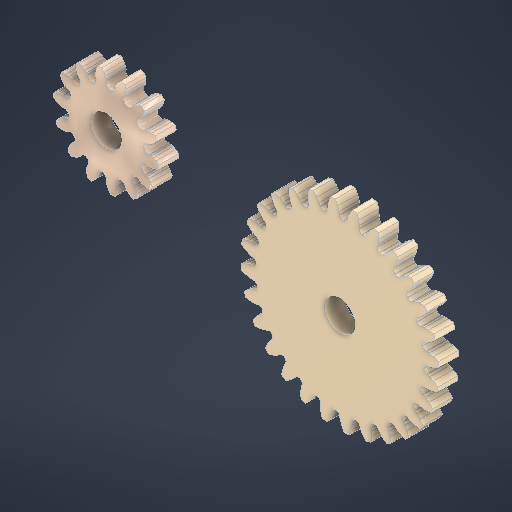
# Autodesk Inventor part: tool_kit
Saved by Autodesk Inventor 2025.3 (Build 293356030, 356C)
## iProperties
Created: 2025-09-03
Part Number: tool_kit
Material: 一般
Document SubType Name: Modeling
Designer: 陳泓任
Density: 1 g/cm^3
Appearance: 一般
Author: 陳泓任
Autodesk Inventor part; units mm, degrees
(part 1 of 2)
ref_plane "YZ Plane" through (0, 0, 0) normal (1, 0, 0) x (0, 1, 0)
ref_plane "XZ Plane" through (0, 0, 0) normal (0, 1, 0) x (-1, 0, 0)
ref_plane "XY Plane" through (0, 0, 0) normal (0, 0, 1) x (1, 0, 0)
sketch "草圖2" plane through (0, 0, 0) normal (0, 0, 1) x (1, 0, 0)
  circle A0 centre (-7.2557, 10.9657) radius 2.34
  arc A1 (-2.6311, 4.4378) -> (-2.6735, 4.985) centre (-7.0202, 4.3731) ccw
  arc A2 (-2.6735, 4.985) -> (-2.7674, 5.4236) centre (-5.8615, 4.5318) ccw
  arc A3 (-2.7674, 5.4236) -> (-2.877, 5.7246) centre (-4.9818, 4.7877) ccw
  arc A4 (-2.877, 5.7246) -> (-2.9667, 5.8946) centre (-4.149, 5.1618) ccw
  arc A5 (-2.9667, 5.8946) -> (-3.0034, 5.9471) centre (-3.4078, 5.6255) ccw
  line L0 (-3.0034, 5.9471) -> (-3.0081, 5.9526)
  arc A6 (-2.1124, 6.8641) -> (-3.0081, 5.9526) centre (-2.6737, 6.5198) ccw
  arc A7 (-2.1124, 6.8641) -> (-2.0593, 6.8294) centre (-1.8035, 7.2782) ccw
  arc A8 (-2.0593, 6.8294) -> (-1.8867, 6.7447) centre (-1.362, 8.0329) ccw
  arc A9 (-1.8867, 6.7447) -> (-1.5826, 6.6441) centre (-1.0129, 8.8764) ccw
  arc A10 (-1.5826, 6.6441) -> (-1.1415, 6.5633) centre (-0.7832, 9.7634) ccw
  arc A11 (-1.1415, 6.5633) -> (-0.5932, 6.5372) centre (-0.659, 10.9263) ccw
  arc A12 (-0.2567, 7.0908) -> (-0.5324, 7.5655) centre (-4.1831, 5.1281) ccw
  arc A13 (-0.5324, 7.5655) -> (-0.8072, 7.9198) centre (-3.208, 5.7739) ccw
  arc A14 (-0.8072, 7.9198) -> (-1.0366, 8.1435) centre (-2.5264, 6.3861) ccw
  arc A15 (-1.0366, 8.1435) -> (-1.1912, 8.2577) centre (-1.9384, 7.0845) ccw
  arc A16 (-1.1912, 8.2577) -> (-1.247, 8.2891) centre (-1.4718, 7.8239) ccw
  line L1 (-1.247, 8.2891) -> (-1.2536, 8.292)
  arc A17 (-0.8422, 9.5019) -> (-1.2536, 8.292) centre (-1.1985, 8.9482) ccw
  arc A18 (-0.8422, 9.5019) -> (-0.7792, 9.4936) centre (-0.7435, 10.009) ccw
  arc A19 (-0.7792, 9.4936) -> (-0.587, 9.4922) centre (-0.6731, 10.8805) ccw
  arc A20 (-0.587, 9.4922) -> (-0.2694, 9.5335) centre (-0.7246, 11.792) ccw
  arc A21 (-0.2694, 9.5335) -> (0.1632, 9.6521) centre (-0.9025, 12.6907) ccw
  arc A22 (0.1632, 9.6521) -> (0.6684, 9.8665) centre (-1.2952, 13.7924) ccw
  arc A23 (0.7314, 10.5113) -> (0.2771, 10.8193) centre (-1.9546, 7.0394) ccw
  arc A24 (0.2771, 10.8193) -> (-0.1243, 11.0193) centre (-1.3562, 8.0443) ccw
  arc A25 (-0.1243, 11.0193) -> (-0.4279, 11.1213) centre (-1.0078, 8.8916) ccw
  arc A26 (-0.4279, 11.1213) -> (-0.6168, 11.1571) centre (-0.781, 9.7759) ccw
  arc A27 (-0.6168, 11.1571) -> (-0.6807, 11.1612) centre (-0.6814, 10.6445) ccw
  line L2 (-0.6807, 11.1612) -> (-0.6879, 11.161)
  arc A28 (-0.8422, 12.4296) -> (-0.6879, 11.161) centre (-0.923, 11.7761) ccw
  arc A29 (-0.8422, 12.4296) -> (-0.7819, 12.4494) centre (-0.9733, 12.9293) ccw
  arc A30 (-0.7819, 12.4494) -> (-0.6081, 12.5316) centre (-1.288, 13.745) ccw
  arc A31 (-0.6081, 12.5316) -> (-0.3398, 12.7066) centre (-1.7299, 14.5439) ccw
  arc A32 (-0.3398, 12.7066) -> (-0.0016, 13.0011) centre (-2.2801, 15.2764) ccw
  arc A33 (-0.0016, 13.0011) -> (0.3606, 13.4135) centre (-3.1119, 16.0986) ccw
  arc A34 (0.1376, 14.0217) -> (-0.4053, 14.1022) centre (-0.776, 9.7283) ccw
  arc A35 (-0.4053, 14.1022) -> (-0.8538, 14.1082) centre (-0.6729, 10.8933) ccw
  arc A36 (-0.8538, 14.1082) -> (-1.1716, 14.0684) centre (-0.7266, 11.8079) ccw
  arc A37 (-1.1716, 14.0684) -> (-1.3573, 14.0187) centre (-0.906, 12.703) ccw
  arc A38 (-1.3573, 14.0187) -> (-1.4167, 13.9946) centre (-1.1931, 13.5288) ccw
  line L3 (-1.4167, 13.9946) -> (-1.4231, 13.9913)
  arc A39 (-2.1125, 15.0673) -> (-1.4231, 13.9913) centre (-1.9017, 14.4435) ccw
  arc A40 (-2.1125, 15.0673) -> (-2.0667, 15.1114) centre (-2.4474, 15.4607) ccw
  arc A41 (-2.0667, 15.1114) -> (-1.9458, 15.2608) centre (-3.0849, 16.059) ccw
  arc A42 (-1.9458, 15.2608) -> (-1.7801, 15.5349) centre (-3.8296, 16.5871) ccw
  arc A43 (-1.7801, 15.5349) -> (-1.6031, 15.947) centre (-4.6432, 17.0083) ccw
  arc A44 (-1.6031, 15.947) -> (-1.4557, 16.4757) centre (-5.7494, 17.3882) ccw
  arc A45 (-1.9205, 16.9269) -> (-2.4446, 16.7638) centre (-0.8808, 12.6622) ccw
  arc A46 (-2.4446, 16.7638) -> (-2.8513, 16.5747) centre (-1.2934, 13.7566) ccw
  arc A47 (-2.8513, 16.5747) -> (-3.1203, 16.4009) centre (-1.7386, 14.5573) ccw
  arc A48 (-3.1203, 16.4009) -> (-3.2661, 16.2756) centre (-2.2886, 15.286) ccw
  arc A49 (-3.2661, 16.2756) -> (-3.3091, 16.2281) centre (-2.9056, 15.9054) ccw
  line L4 (-3.3091, 16.2281) -> (-3.3134, 16.2223)
  arc A50 (-4.4014, 16.8927) -> (-3.3134, 16.2223) centre (-3.9409, 16.4221) ccw
  arc A51 (-4.4014, 16.8927) -> (-4.3793, 16.9522) centre (-4.8739, 17.1018) ccw
  arc A52 (-4.3793, 16.9522) -> (-4.3352, 17.1393) centre (-5.7078, 17.3643) ccw
  arc A53 (-4.3352, 17.1393) -> (-4.3048, 17.4582) centre (-6.6079, 17.5169) ccw
  arc A54 (-4.3048, 17.4582) -> (-4.3242, 17.9062) centre (-7.5237, 17.5434) ccw
  arc A55 (-4.3242, 17.9062) -> (-4.4207, 18.4466) centre (-8.6852, 17.4058) ccw
  arc A56 (-5.0353, 18.6514) -> (-5.4368, 18.2771) centre (-2.2482, 15.2602) ccw
  arc A57 (-5.4368, 18.2771) -> (-5.7211, 17.9302) centre (-3.0947, 16.0672) ccw
  arc A58 (-5.7211, 17.9302) -> (-5.8881, 17.6569) centre (-3.8433, 16.5954) ccw
  arc A59 (-5.8881, 17.6569) -> (-5.965, 17.4808) centre (-4.655, 17.0133) ccw
  arc A60 (-5.965, 17.4808) -> (-5.9832, 17.4193) centre (-5.4796, 17.3037) ccw
  line L5 (-5.9832, 17.4193) -> (-5.9846, 17.4123)
  arc A61 (-7.2557, 17.5441) -> (-5.9846, 17.4123) centre (-6.6366, 17.32) ccw
  arc A62 (-7.2557, 17.5441) -> (-7.2616, 17.6074) centre (-7.7721, 17.5275) ccw
  arc A63 (-7.2616, 17.6074) -> (-7.3031, 17.7951) centre (-8.6374, 17.4022) ccw
  arc A64 (-7.3031, 17.7951) -> (-7.414, 18.0956) centre (-9.5146, 17.1492) ccw
  arc A65 (-7.414, 18.0956) -> (-7.6259, 18.4908) centre (-10.3512, 16.7757) ccw
  arc A66 (-7.6259, 18.4908) -> (-7.9473, 18.9358) centre (-11.3378, 16.1478) ccw
  arc A67 (-8.5899, 18.8537) -> (-8.7892, 18.3422) centre (-4.6074, 17.0076) ccw
  arc A68 (-8.7892, 18.3422) -> (-8.8949, 17.9064) centre (-5.7202, 17.3673) ccw
  arc A69 (-8.8949, 17.9064) -> (-8.9267, 17.5876) centre (-6.6239, 17.5185) ccw
  arc A70 (-8.9267, 17.5876) -> (-8.9196, 17.3956) centre (-7.5365, 17.5428) ccw
  arc A71 (-8.9196, 17.3956) -> (-8.9093, 17.3323) centre (-8.4055, 17.4466) ccw
  line L6 (-8.9093, 17.3323) -> (-8.9075, 17.3253)
  arc A72 (-10.11, 16.8927) -> (-8.9075, 17.3253) centre (-9.4549, 16.9593) ccw
  arc A73 (-10.11, 16.8927) -> (-10.1428, 16.947) centre (-10.568, 16.6536) ccw
  arc A74 (-10.1428, 16.947) -> (-10.2615, 17.0982) centre (-11.2932, 16.1653) ccw
  arc A75 (-10.2615, 17.0982) -> (-10.4919, 17.3208) centre (-11.9738, 15.5567) ccw
  arc A76 (-10.4919, 17.3208) -> (-10.8543, 17.585) centre (-12.5655, 14.8573) ccw
  arc A77 (-10.8543, 17.585) -> (-11.3369, 17.8464) centre (-13.182, 13.8634) ccw
  arc A78 (-11.8803, 17.4936) -> (-11.8379, 16.9464) centre (-7.4911, 17.5583) ccw
  arc A79 (-11.8379, 16.9464) -> (-11.744, 16.5078) centre (-8.6499, 17.3996) ccw
  arc A80 (-11.744, 16.5078) -> (-11.6344, 16.2068) centre (-9.5296, 17.1437) ccw
  arc A81 (-11.6344, 16.2068) -> (-11.5446, 16.0368) centre (-10.3624, 16.7696) ccw
  arc A82 (-11.5446, 16.0368) -> (-11.5079, 15.9843) centre (-11.1036, 16.3059) ccw
  line L7 (-11.5079, 15.9843) -> (-11.5033, 15.9788)
  arc A83 (-12.3989, 15.0673) -> (-11.5033, 15.9788) centre (-11.8376, 15.4116) ccw
  arc A84 (-12.3989, 15.0673) -> (-12.4521, 15.1021) centre (-12.7079, 14.6532) ccw
  arc A85 (-12.4521, 15.1021) -> (-12.6246, 15.1867) centre (-13.1494, 13.8985) ccw
  arc A86 (-12.6246, 15.1867) -> (-12.9288, 15.2873) centre (-13.4985, 13.055) ccw
  arc A87 (-12.9288, 15.2873) -> (-13.3699, 15.3681) centre (-13.7281, 12.168) ccw
  arc A88 (-13.3699, 15.3681) -> (-13.9181, 15.3942) centre (-13.8524, 11.0051) ccw
  arc A89 (-14.2546, 14.8406) -> (-13.979, 14.366) centre (-10.3282, 16.8033) ccw
  arc A90 (-13.979, 14.366) -> (-13.7041, 14.0116) centre (-11.3033, 16.1575) ccw
  arc A91 (-13.7041, 14.0116) -> (-13.4748, 13.7879) centre (-11.9849, 15.5453) ccw
  arc A92 (-13.4748, 13.7879) -> (-13.3202, 13.6737) centre (-12.573, 14.8469) ccw
  arc A93 (-13.3202, 13.6737) -> (-13.2643, 13.6423) centre (-13.0395, 14.1075) ccw
  line L8 (-13.2643, 13.6423) -> (-13.2578, 13.6394)
  arc A94 (-13.6692, 12.4295) -> (-13.2578, 13.6394) centre (-13.3129, 12.9832) ccw
  arc A95 (-13.6692, 12.4295) -> (-13.7321, 12.4378) centre (-13.7679, 11.9224) ccw
  arc A96 (-13.7321, 12.4378) -> (-13.9243, 12.4392) centre (-13.8382, 11.0509) ccw
  arc A97 (-13.9243, 12.4392) -> (-14.242, 12.3979) centre (-13.7868, 10.1394) ccw
  arc A98 (-14.242, 12.3979) -> (-14.6745, 12.2793) centre (-13.6088, 9.2407) ccw
  arc A99 (-14.6745, 12.2793) -> (-15.1798, 12.0649) centre (-13.2162, 8.139) ccw
  arc A100 (-15.231, 11.5938) -> (-15.2428, 11.4201) centre (-7.2557, 10.9657) ccw
  arc A101 (-15.2428, 11.4201) -> (-14.7885, 11.1121) centre (-12.5568, 14.892) ccw
  arc A102 (-14.7885, 11.1121) -> (-14.3871, 10.9121) centre (-13.1551, 13.8871) ccw
  arc A103 (-14.3871, 10.9121) -> (-14.0834, 10.8101) centre (-13.5036, 13.0398) ccw
  arc A104 (-14.0834, 10.8101) -> (-13.8946, 10.7743) centre (-13.7304, 12.1555) ccw
  arc A105 (-13.8946, 10.7743) -> (-13.8306, 10.7702) centre (-13.83, 11.2869) ccw
  line L9 (-13.8306, 10.7702) -> (-13.8235, 10.7704)
  arc A106 (-13.6692, 9.5018) -> (-13.8235, 10.7704) centre (-13.5884, 10.1553) ccw
  arc A107 (-13.6692, 9.5018) -> (-13.7295, 9.482) centre (-13.5381, 9.0021) ccw
  arc A108 (-13.7295, 9.482) -> (-13.9033, 9.3998) centre (-13.2233, 8.1864) ccw
  arc A109 (-13.9033, 9.3998) -> (-14.1715, 9.2248) centre (-12.7815, 7.3875) ccw
  arc A110 (-14.1715, 9.2248) -> (-14.5098, 8.9303) centre (-12.2312, 6.655) ccw
  arc A111 (-14.5098, 8.9303) -> (-14.872, 8.5179) centre (-11.3995, 5.8328) ccw
  arc A112 (-14.649, 7.9097) -> (-14.106, 7.8292) centre (-13.7354, 12.2032) ccw
  arc A113 (-14.106, 7.8292) -> (-13.6576, 7.8232) centre (-13.8385, 11.0382) ccw
  arc A114 (-13.6576, 7.8232) -> (-13.3397, 7.8631) centre (-13.7848, 10.1235) ccw
  arc A115 (-13.3397, 7.8631) -> (-13.1541, 7.9127) centre (-13.6054, 9.2284) ccw
  arc A116 (-13.1541, 7.9127) -> (-13.0947, 7.9368) centre (-13.3182, 8.4026) ccw
  line L10 (-13.0947, 7.9368) -> (-13.0883, 7.9401)
  arc A117 (-12.3989, 6.8641) -> (-13.0883, 7.9401) centre (-12.6097, 7.4879) ccw
  arc A118 (-12.3989, 6.8641) -> (-12.4446, 6.82) centre (-12.0639, 6.4707) ccw
  arc A119 (-12.4446, 6.82) -> (-12.5655, 6.6706) centre (-11.4265, 5.8724) ccw
  arc A120 (-12.5655, 6.6706) -> (-12.7313, 6.3965) centre (-10.6817, 5.3443) ccw
  arc A121 (-12.7313, 6.3965) -> (-12.9083, 5.9844) centre (-9.8681, 4.9231) ccw
  arc A122 (-12.9083, 5.9844) -> (-13.0557, 5.4557) centre (-8.762, 4.5432) ccw
  arc A123 (-12.5908, 5.0045) -> (-12.0668, 5.1676) centre (-13.6306, 9.2692) ccw
  arc A124 (-12.0668, 5.1676) -> (-11.6601, 5.3567) centre (-13.218, 8.1748) ccw
  arc A125 (-11.6601, 5.3567) -> (-11.391, 5.5305) centre (-12.7728, 7.3741) ccw
  arc A126 (-11.391, 5.5305) -> (-11.2453, 5.6558) centre (-12.2228, 6.6454) ccw
  arc A127 (-11.2453, 5.6558) -> (-11.2022, 5.7033) centre (-11.6058, 6.026) ccw
  line L11 (-11.2022, 5.7033) -> (-11.1979, 5.7091)
  arc A128 (-10.1099, 5.0387) -> (-11.1979, 5.7091) centre (-10.5705, 5.5093) ccw
  arc A129 (-10.1099, 5.0387) -> (-10.132, 4.9792) centre (-9.6375, 4.8296) ccw
  arc A130 (-10.132, 4.9792) -> (-10.1761, 4.7921) centre (-8.8035, 4.5672) ccw
  arc A131 (-10.1761, 4.7921) -> (-10.2066, 4.4732) centre (-7.9034, 4.4145) ccw
  arc A132 (-10.2066, 4.4732) -> (-10.1872, 4.0252) centre (-6.9876, 4.388) ccw
  arc A133 (-10.1872, 4.0252) -> (-10.0906, 3.4849) centre (-5.8262, 4.5256) ccw
  arc A134 (-9.476, 3.28) -> (-9.0746, 3.6543) centre (-12.2632, 6.6712) ccw
  arc A135 (-9.0746, 3.6543) -> (-8.7903, 4.0012) centre (-11.4166, 5.8642) ccw
  arc A136 (-8.7903, 4.0012) -> (-8.6233, 4.2745) centre (-10.6681, 5.336) ccw
  arc A137 (-8.6233, 4.2745) -> (-8.5463, 4.4507) centre (-9.8564, 4.9181) ccw
  arc A138 (-8.5463, 4.4507) -> (-8.5282, 4.5121) centre (-9.0317, 4.6277) ccw
  line L12 (-8.5282, 4.5121) -> (-8.5268, 4.5191)
  arc A139 (-7.2557, 4.3873) -> (-8.5268, 4.5191) centre (-7.8748, 4.6114) ccw
  arc A140 (-7.2557, 4.3873) -> (-7.2497, 4.324) centre (-6.7393, 4.4039) ccw
  arc A141 (-7.2497, 4.324) -> (-7.2083, 4.1364) centre (-5.874, 4.5292) ccw
  arc A142 (-7.2083, 4.1364) -> (-7.0973, 3.8358) centre (-4.9968, 4.7822) ccw
  arc A143 (-7.0973, 3.8358) -> (-6.8855, 3.4406) centre (-4.1602, 5.1557) ccw
  arc A144 (-6.8855, 3.4406) -> (-6.5641, 2.9957) centre (-3.1735, 5.7836) ccw
  arc A145 (-5.9214, 3.0778) -> (-5.7222, 3.5892) centre (-9.904, 4.9238) ccw
  arc A146 (-5.7222, 3.5892) -> (-5.6165, 4.025) centre (-8.7911, 4.5641) ccw
  arc A147 (-5.6165, 4.025) -> (-5.5847, 4.3438) centre (-7.8875, 4.4129) ccw
  arc A148 (-5.5847, 4.3438) -> (-5.5918, 4.5359) centre (-6.9749, 4.3886) ccw
  arc A149 (-5.5918, 4.5359) -> (-5.602, 4.5991) centre (-6.1059, 4.4848) ccw
  line L13 (-5.602, 4.5991) -> (-5.6038, 4.6061)
  arc A150 (-4.4014, 5.0387) -> (-5.6038, 4.6061) centre (-5.0565, 4.9721) ccw
  arc A151 (-4.4014, 5.0387) -> (-4.3686, 4.9844) centre (-3.9433, 5.2778) ccw
  arc A152 (-4.3686, 4.9844) -> (-4.2499, 4.8332) centre (-3.2182, 5.7661) ccw
  arc A153 (-4.2499, 4.8332) -> (-4.0195, 4.6106) centre (-2.5376, 6.3747) ccw
  arc A154 (-4.0195, 4.6106) -> (-3.6571, 4.3464) centre (-1.9459, 7.0741) ccw
  arc A155 (-3.6571, 4.3464) -> (-3.1745, 4.085) centre (-1.3294, 8.068) ccw
  circle A156 centre (28.1558, 4.4199) radius 2.34
  arc A157 (31.0202, 18.3926) -> (30.8085, 19.1835) centre (24.7058, 17.1262) ccw
  arc A158 (31.1028, 17.7572) -> (31.0202, 18.3926) centre (26.5033, 17.4821) ccw
  arc A159 (31.1, 17.3728) -> (31.1028, 17.7572) centre (28.3263, 17.585) ccw
  arc A160 (31.0898, 17.2827) -> (31.1, 17.3728) centre (30.0691, 17.4444) ccw
  arc A161 (31.0898, 17.2827) -> (31.4895, 16.7266) centre (31.6154, 17.2389) ccw
  line L14 (31.4895, 16.7266) -> (31.4898, 16.728)
  arc A162 (31.4898, 16.728) -> (31.5032, 16.7235) centre (31.6675, 17.2247) ccw
  arc A163 (31.5032, 16.7235) -> (31.517, 16.7206) centre (31.6154, 17.2389) ccw
  line L15 (31.517, 16.7206) -> (31.5166, 16.7192)
  arc A164 (31.5166, 16.7192) -> (32.143, 16.9961) centre (31.6675, 17.2247) ccw
  arc A165 (32.1798, 17.0791) -> (32.143, 16.9961) centre (33.1048, 16.6184) ccw
  arc A166 (32.3722, 17.4119) -> (32.1798, 17.0791) centre (34.6787, 15.8567) ccw
  arc A167 (32.7653, 17.9178) -> (32.3722, 17.4119) centre (36.1983, 14.8444) ccw
  arc A168 (33.3485, 18.4924) -> (32.7653, 17.9178) centre (37.5677, 13.6269) ccw
  arc A169 (34.0576, 17.4049) -> (34.0272, 18.2231) centre (27.6197, 17.5754) ccw
  arc A170 (33.9967, 16.7671) -> (34.0576, 17.4049) centre (29.4513, 17.5224) ccw
  arc A171 (33.9085, 16.3929) -> (33.9967, 16.7671) centre (31.2515, 17.217) ccw
  arc A172 (33.8784, 16.3073) -> (33.9085, 16.3929) centre (32.9194, 16.692) ccw
  arc A173 (33.8784, 16.3073) -> (34.1444, 15.6763) centre (34.3812, 16.1476) ccw
  line L16 (34.1444, 15.6763) -> (34.1451, 15.6775)
  arc A174 (34.1451, 15.6775) -> (34.1571, 15.6701) centre (34.4288, 16.1222) ccw
  arc A175 (34.1571, 15.6701) -> (34.1699, 15.6643) centre (34.3812, 16.1476) ccw
  line L17 (34.1699, 15.6643) -> (34.1692, 15.663)
  arc A176 (34.1692, 15.663) -> (34.8415, 15.7936) centre (34.4288, 16.1222) ccw
  arc A177 (34.8958, 15.8663) -> (34.8415, 15.7936) centre (35.6952, 15.2113) ccw
  arc A178 (35.1574, 16.1479) -> (34.8958, 15.8663) centre (37.0601, 14.1185) ccw
  arc A179 (35.6533, 16.5537) -> (35.1574, 16.1479) centre (38.3163, 12.7934) ccw
  arc A180 (36.3498, 16.9841) -> (35.6533, 16.5537) centre (39.3805, 11.3017) ccw
  arc A181 (36.799, 15.7661) -> (36.9514, 16.5705) centre (30.5605, 17.3648) ccw
  arc A182 (36.5978, 15.1578) -> (36.799, 15.7661) centre (32.3344, 16.9056) ccw
  arc A183 (36.4285, 14.8127) -> (36.5978, 15.1578) centre (34.0215, 16.2073) ccw
  arc A184 (36.3802, 14.7359) -> (36.4285, 14.8127) centre (35.5308, 15.3244) ccw
  arc A185 (36.3802, 14.7359) -> (36.499, 14.0615) centre (36.8348, 14.4683) ccw
  line L18 (36.499, 14.0615) -> (36.5, 14.0626)
  arc A186 (36.5, 14.0626) -> (36.51, 14.0526) centre (36.8756, 14.4329) ccw
  arc A187 (36.51, 14.0526) -> (36.5212, 14.0441) centre (36.8348, 14.4683) ccw
  line L19 (36.5212, 14.0441) -> (36.5203, 14.043)
  arc A188 (36.5203, 14.043) -> (37.2047, 14.0207) centre (36.8756, 14.4329) ccw
  arc A189 (37.2739, 14.0795) -> (37.2047, 14.0207) centre (37.9075, 13.2631) ccw
  arc A190 (37.5916, 14.2959) -> (37.2739, 14.0795) centre (38.995, 11.8939) ccw
  arc A191 (38.1653, 14.5811) -> (37.5916, 14.2959) centre (39.9249, 10.3226) ccw
  arc A192 (38.9401, 14.8458) -> (38.1653, 14.5811) centre (40.6304, 8.6315) ccw
  arc A193 (39.1071, 13.5583) -> (39.4347, 14.3087) centre (33.3807, 16.5052) ccw
  arc A194 (38.7755, 13.0101) -> (39.1071, 13.5583) centre (35.008, 15.6627) ccw
  arc A195 (38.5337, 12.7112) -> (38.7755, 13.0101) centre (36.4974, 14.6065) ccw
  arc A196 (38.4695, 12.6471) -> (38.5337, 12.7112) centre (37.7723, 13.4099) ccw
  arc A197 (38.4695, 12.6471) -> (38.4353, 11.9632) centre (38.8531, 12.2851) ccw
  line L20 (38.4353, 11.9632) -> (38.4364, 11.9641)
  arc A198 (38.4364, 11.9641) -> (38.444, 11.9522) centre (38.885, 12.2416) ccw
  arc A199 (38.444, 11.9522) -> (38.4531, 11.9413) centre (38.8531, 12.2851) ccw
  line L21 (38.4531, 11.9413) -> (38.4519, 11.9405)
  arc A200 (38.4519, 11.9405) -> (39.1142, 11.7665) centre (38.885, 12.2416) ccw
  arc A201 (39.1947, 11.8083) -> (39.1142, 11.7665) centre (39.6308, 10.8715) ccw
  arc A202 (39.5527, 11.9486) -> (39.1947, 11.8083) centre (40.3864, 9.2946) ccw
  arc A203 (40.1754, 12.099) -> (39.5527, 11.9486) centre (40.9433, 7.5557) ccw
  arc A204 (40.9897, 12.1847) -> (40.1754, 12.099) centre (41.2548, 5.75) ccw
  arc A205 (40.866, 10.8923) -> (41.3523, 11.551) centre (35.9389, 15.0395) ccw
  arc A206 (40.4208, 10.4316) -> (40.866, 10.8923) centre (37.3379, 13.8561) ccw
  arc A207 (40.1185, 10.1941) -> (40.4208, 10.4316) centre (38.555, 12.495) ccw
  arc A208 (40.0416, 10.1459) -> (40.1185, 10.1941) centre (39.5317, 11.0446) ccw
  arc A209 (40.0416, 10.1459) -> (39.8561, 9.4867) centre (40.3351, 9.7076) ccw
  line L22 (39.8561, 9.4867) -> (39.8574, 9.4873)
  arc A210 (39.8574, 9.4873) -> (39.8622, 9.474) centre (40.3565, 9.658) ccw
  arc A211 (39.8622, 9.474) -> (39.8686, 9.4614) centre (40.3351, 9.7076) ccw
  line L23 (39.8686, 9.4614) -> (39.8673, 9.4608)
  arc A212 (39.8673, 9.4608) -> (40.4742, 9.1438) centre (40.3565, 9.658) ccw
  arc A213 (40.5621, 9.1667) -> (40.4742, 9.1438) centre (40.7787, 8.1563) ccw
  arc A214 (40.9422, 9.2238) -> (40.5621, 9.1667) centre (41.1644, 6.4508) ccw
  arc A215 (41.5828, 9.2319) -> (40.9422, 9.2238) centre (41.3204, 4.6316) ccw
  arc A216 (42.3958, 9.1342) -> (41.5828, 9.2319) centre (41.2224, 2.8019) ccw
  arc A217 (41.9875, 7.9017) -> (42.6083, 8.4357) centre (38.1069, 13.0414) ccw
  arc A218 (41.451, 7.5516) -> (41.9875, 7.9017) centre (39.2074, 11.5763) ccw
  arc A219 (41.1034, 7.3874) -> (41.451, 7.5516) centre (40.0911, 9.9785) ccw
  arc A220 (41.0178, 7.3575) -> (41.1034, 7.3874) centre (40.7206, 8.3472) ccw
  arc A221 (41.0178, 7.3575) -> (40.6902, 6.7561) centre (41.2064, 6.8648) ccw
  line L24 (40.6902, 6.7561) -> (40.6916, 6.7564)
  arc A222 (40.6916, 6.7564) -> (40.6933, 6.7423) centre (41.2162, 6.8117) ccw
  arc A223 (40.6933, 6.7423) -> (40.6968, 6.7287) centre (41.2064, 6.8648) ccw
  line L25 (40.6968, 6.7287) -> (40.6953, 6.7284)
  arc A224 (40.6953, 6.7284) -> (41.2166, 6.2842) centre (41.2162, 6.8117) ccw
  arc A225 (41.3073, 6.287) -> (41.2166, 6.2842) centre (41.2936, 5.2538) ccw
  arc A226 (41.6906, 6.2581) -> (41.3073, 6.287) centre (41.2902, 3.5052) ccw
  arc A227 (42.3169, 6.1234) -> (41.6906, 6.2581) centre (41.0375, 1.6969) ccw
  arc A228 (43.0878, 5.8473) -> (42.3169, 6.1234) centre (40.5347, -0.0652) ccw
  arc A229 (42.4155, 4.7366) -> (43.1395, 5.119) centre (39.7758, 10.6109) ccw
  arc A230 (41.8145, 4.5147) -> (42.4155, 4.7366) centre (40.5228, 8.9377) ccw
  arc A231 (41.4391, 4.4318) -> (41.8145, 4.5147) centre (41.0288, 7.1833) ccw
  arc A232 (41.3489, 4.4218) -> (41.4391, 4.4318) centre (41.2795, 5.4528) ccw
  arc A233 (41.3489, 4.4218) -> (40.8958, 3.9084) centre (41.4232, 3.8995) ccw
  line L26 (40.8958, 3.9084) -> (40.8972, 3.9083)
  arc A234 (40.8972, 3.9083) -> (40.8957, 3.8943) centre (41.421, 3.8456) ccw
  arc A235 (40.8957, 3.8943) -> (40.8961, 3.8801) centre (41.4232, 3.8995) ccw
  line L27 (40.8961, 3.8801) -> (40.8946, 3.8802)
  arc A236 (40.8946, 3.8802) -> (41.3039, 3.3312) centre (41.421, 3.8456) ccw
  arc A237 (41.393, 3.3138) -> (41.3039, 3.3312) centre (41.1498, 2.3094) ccw
  arc A238 (41.7603, 3.2003) -> (41.393, 3.3138) centre (40.7574, 0.6055) ccw
  arc A239 (42.341, 2.9296) -> (41.7603, 3.2003) centre (40.1086, -1.1013) ccw
  arc A240 (43.031, 2.4888) -> (42.341, 2.9296) centre (39.2263, -2.7073) ccw
  arc A241 (42.1285, 1.5556) -> (42.9194, 1.7673) centre (40.8621, 7.87) ccw
  arc A242 (41.4931, 1.473) -> (42.1285, 1.5556) centre (41.218, 6.0725) ccw
  arc A243 (41.1087, 1.4757) -> (41.4931, 1.473) centre (41.3209, 4.2495) ccw
  arc A244 (41.0186, 1.486) -> (41.1087, 1.4757) centre (41.1802, 2.5066) ccw
  arc A245 (41.0186, 1.486) -> (40.4625, 1.0863) centre (40.9748, 0.9603) ccw
  line L28 (40.4625, 1.0863) -> (40.4639, 1.0859)
  arc A246 (40.4639, 1.0859) -> (40.4593, 1.0725) centre (40.9606, 0.9082) ccw
  arc A247 (40.4593, 1.0725) -> (40.4565, 1.0587) centre (40.9748, 0.9603) ccw
  line L29 (40.4565, 1.0587) -> (40.4551, 1.0591)
  arc A248 (40.4551, 1.0591) -> (40.732, 0.4328) centre (40.9606, 0.9082) ccw
  arc A249 (40.815, 0.3959) -> (40.732, 0.4328) centre (40.3543, -0.5291) ccw
  arc A250 (41.1478, 0.2036) -> (40.815, 0.3959) centre (39.5926, -2.103) ccw
  arc A251 (41.6537, -0.1895) -> (41.1478, 0.2036) centre (38.5803, -3.6226) ccw
  arc A252 (42.2283, -0.7728) -> (41.6537, -0.1895) centre (37.3628, -4.992) ccw
  arc A253 (41.1408, -1.4818) -> (41.959, -1.4514) centre (41.3113, 4.956) ccw
  arc A254 (40.503, -1.421) -> (41.1408, -1.4818) centre (41.2583, 3.1244) ccw
  arc A255 (40.1288, -1.3328) -> (40.503, -1.421) centre (40.9529, 1.3242) ccw
  arc A256 (40.0432, -1.3027) -> (40.1288, -1.3328) centre (40.4279, -0.3436) ccw
  arc A257 (40.0432, -1.3027) -> (39.4122, -1.5686) centre (39.8835, -1.8054) ccw
  line L30 (39.4122, -1.5686) -> (39.4134, -1.5693)
  arc A258 (39.4134, -1.5693) -> (39.406, -1.5813) centre (39.8581, -1.8531) ccw
  arc A259 (39.406, -1.5813) -> (39.4002, -1.5942) centre (39.8835, -1.8054) ccw
  line L31 (39.4002, -1.5942) -> (39.3989, -1.5935)
  arc A260 (39.3989, -1.5935) -> (39.5295, -2.2657) centre (39.8581, -1.8531) ccw
  arc A261 (39.6022, -2.3201) -> (39.5295, -2.2657) centre (38.9472, -3.1194) ccw
  arc A262 (39.8838, -2.5817) -> (39.6022, -2.3201) centre (37.8544, -4.4844) ccw
  arc A263 (40.2896, -3.0775) -> (39.8838, -2.5817) centre (36.5293, -5.7406) ccw
  arc A264 (40.72, -3.774) -> (40.2896, -3.0775) centre (35.0376, -6.8048) ccw
  arc A265 (39.502, -4.2233) -> (40.3064, -4.3757) centre (41.1007, 2.0152) ccw
  arc A266 (38.8937, -4.0221) -> (39.502, -4.2233) centre (40.6415, 0.2413) ccw
  arc A267 (38.5486, -3.8528) -> (38.8937, -4.0221) centre (39.9432, -1.4458) ccw
  arc A268 (38.4718, -3.8044) -> (38.5486, -3.8528) centre (39.0603, -2.955) ccw
  arc A269 (38.4718, -3.8044) -> (37.7974, -3.9233) centre (38.2042, -4.259) ccw
  line L32 (37.7974, -3.9233) -> (37.7985, -3.9242)
  arc A270 (37.7985, -3.9242) -> (37.7885, -3.9343) centre (38.1688, -4.2998) ccw
  arc A271 (37.7885, -3.9343) -> (37.78, -3.9455) centre (38.2042, -4.259) ccw
  line L33 (37.78, -3.9455) -> (37.7789, -3.9446)
  arc A272 (37.7789, -3.9446) -> (37.7566, -4.629) centre (38.1688, -4.2998) ccw
  arc A273 (37.8154, -4.6982) -> (37.7566, -4.629) centre (36.999, -5.3317) ccw
  arc A274 (38.0318, -5.0159) -> (37.8154, -4.6982) centre (35.6298, -6.4193) ccw
  arc A275 (38.317, -5.5896) -> (38.0318, -5.0159) centre (34.0585, -7.3491) ccw
  arc A276 (38.5817, -6.3644) -> (38.317, -5.5896) centre (32.3674, -8.0547) ccw
  arc A277 (37.2942, -6.5313) -> (38.0446, -6.8589) centre (40.2411, -0.805) ccw
  arc A278 (36.746, -6.1998) -> (37.2942, -6.5313) centre (39.3986, -2.4322) ccw
  arc A279 (36.4471, -5.958) -> (36.746, -6.1998) centre (38.3424, -3.9216) ccw
  arc A280 (36.383, -5.8937) -> (36.4471, -5.958) centre (37.1458, -5.1966) ccw
  arc A281 (36.383, -5.8937) -> (35.6991, -5.8595) centre (36.021, -6.2774) ccw
  line L34 (35.6991, -5.8595) -> (35.7, -5.8607)
  arc A282 (35.7, -5.8607) -> (35.6881, -5.8683) centre (35.9775, -6.3093) ccw
  arc A283 (35.6881, -5.8683) -> (35.6772, -5.8773) centre (36.021, -6.2774) ccw
  line L35 (35.6772, -5.8773) -> (35.6764, -5.8762)
  arc A284 (35.6764, -5.8762) -> (35.5024, -6.5385) centre (35.9775, -6.3093) ccw
  arc A285 (35.5442, -6.619) -> (35.5024, -6.5385) centre (34.6074, -7.055) ccw
  arc A286 (35.6845, -6.9769) -> (35.5442, -6.619) centre (33.0305, -7.8106) ccw
  arc A287 (35.8349, -7.5997) -> (35.6845, -6.9769) centre (31.2916, -8.3675) ccw
  arc A288 (35.9206, -8.414) -> (35.8349, -7.5997) centre (29.4859, -8.6791) ccw
  arc A289 (34.6282, -8.2902) -> (35.2868, -8.7766) centre (38.7754, -3.3632) ccw
  arc A290 (34.1675, -7.845) -> (34.6282, -8.2902) centre (37.592, -4.7622) ccw
  arc A291 (33.93, -7.5428) -> (34.1675, -7.845) centre (36.2309, -5.9792) ccw
  arc A292 (33.8818, -7.4659) -> (33.93, -7.5428) centre (34.7805, -6.9559) ccw
  arc A293 (33.8818, -7.4659) -> (33.2226, -7.2803) centre (33.4435, -7.7594) ccw
  line L36 (33.2226, -7.2803) -> (33.2232, -7.2817)
  arc A294 (33.2232, -7.2817) -> (33.2099, -7.2864) centre (33.3939, -7.7808) ccw
  arc A295 (33.2099, -7.2864) -> (33.1973, -7.2928) centre (33.4435, -7.7594) ccw
  line L37 (33.1973, -7.2928) -> (33.1967, -7.2915)
  arc A296 (33.1967, -7.2915) -> (32.8797, -7.8985) centre (33.3939, -7.7808) ccw
  arc A297 (32.9026, -7.9863) -> (32.8797, -7.8985) centre (31.8922, -8.2029) ccw
  arc A298 (32.9597, -8.3665) -> (32.9026, -7.9863) centre (30.1867, -8.5887) ccw
  arc A299 (32.9678, -9.0071) -> (32.9597, -8.3665) centre (28.3675, -8.7447) ccw
  arc A300 (32.8701, -9.82) -> (32.9678, -9.0071) centre (26.5378, -8.6466) ccw
  arc A301 (31.6376, -9.4118) -> (32.1716, -10.0325) centre (36.7773, -5.5311) ccw
  arc A302 (31.2875, -8.8752) -> (31.6376, -9.4118) centre (35.3122, -6.6317) ccw
  arc A303 (31.1232, -8.5277) -> (31.2875, -8.8752) centre (33.7144, -7.5154) ccw
  arc A304 (31.0934, -8.442) -> (31.1232, -8.5277) centre (32.0831, -8.1448) ccw
  arc A305 (31.0934, -8.442) -> (30.492, -8.1145) centre (30.6007, -8.6306) ccw
  line L38 (30.492, -8.1145) -> (30.4923, -8.1159)
  arc A306 (30.4923, -8.1159) -> (30.4782, -8.1175) centre (30.5476, -8.6405) ccw
  arc A307 (30.4782, -8.1175) -> (30.4646, -8.121) centre (30.6007, -8.6306) ccw
  line L39 (30.4646, -8.121) -> (30.4643, -8.1196)
  arc A308 (30.4643, -8.1196) -> (30.0201, -8.6408) centre (30.5476, -8.6405) ccw
  arc A309 (30.0229, -8.7315) -> (30.0201, -8.6408) centre (28.9897, -8.7179) ccw
  arc A310 (29.994, -9.1148) -> (30.0229, -8.7315) centre (27.2411, -8.7145) ccw
  arc A311 (29.8593, -9.7412) -> (29.994, -9.1148) centre (25.4328, -8.4617) ccw
  arc A312 (29.5832, -10.512) -> (29.8593, -9.7412) centre (23.6707, -7.959) ccw
  arc A313 (28.4725, -9.8398) -> (28.8549, -10.5638) centre (34.3468, -7.2001) ccw
  arc A314 (28.2506, -9.2388) -> (28.4725, -9.8398) centre (32.6736, -7.9471) ccw
  arc A315 (28.1677, -8.8634) -> (28.2506, -9.2388) centre (30.9192, -8.453) ccw
  arc A316 (28.1577, -8.7732) -> (28.1677, -8.8634) centre (29.1887, -8.7037) ccw
  arc A317 (28.1577, -8.7732) -> (27.6443, -8.32) centre (27.6354, -8.8475) ccw
  line L40 (27.6443, -8.32) -> (27.6442, -8.3215)
  arc A318 (27.6442, -8.3215) -> (27.6302, -8.32) centre (27.5815, -8.8452) ccw
  arc A319 (27.6302, -8.32) -> (27.616, -8.3203) centre (27.6354, -8.8475) ccw
  line L41 (27.616, -8.3203) -> (27.6161, -8.3189)
  arc A320 (27.6161, -8.3189) -> (27.0671, -8.7282) centre (27.5815, -8.8452) ccw
  arc A321 (27.0496, -8.8173) -> (27.0671, -8.7282) centre (26.0453, -8.574) ccw
  arc A322 (26.9362, -9.1845) -> (27.0496, -8.8173) centre (24.3414, -8.1816) ccw
  arc A323 (26.6655, -9.7652) -> (26.9362, -9.1845) centre (22.6346, -7.5328) ccw
  arc A324 (26.2247, -10.4553) -> (26.6655, -9.7652) centre (21.0286, -6.6506) ccw
  arc A325 (25.2915, -9.5527) -> (25.5032, -10.3437) centre (31.6059, -8.2864) ccw
  arc A326 (25.2089, -8.9174) -> (25.2915, -9.5527) centre (29.8084, -8.6423) ccw
  arc A327 (25.2116, -8.533) -> (25.2089, -8.9174) centre (27.9854, -8.7452) ccw
  arc A328 (25.2219, -8.4428) -> (25.2116, -8.533) centre (26.2425, -8.6045) ccw
  arc A329 (25.2219, -8.4428) -> (24.8222, -7.8868) centre (24.6962, -8.399) ccw
  line L42 (24.8222, -7.8868) -> (24.8218, -7.8882)
  arc A330 (24.8218, -7.8882) -> (24.8084, -7.8836) centre (24.6441, -8.3849) ccw
  arc A331 (24.8084, -7.8836) -> (24.7946, -7.8808) centre (24.6962, -8.399) ccw
  line L43 (24.7946, -7.8808) -> (24.795, -7.8794)
  arc A332 (24.795, -7.8794) -> (24.1687, -8.1563) centre (24.6441, -8.3849) ccw
  arc A333 (24.1318, -8.2392) -> (24.1687, -8.1563) centre (23.2068, -7.7786) ccw
  arc A334 (23.9395, -8.572) -> (24.1318, -8.2392) centre (21.6329, -7.0169) ccw
  arc A335 (23.5464, -9.0779) -> (23.9395, -8.572) centre (20.1133, -6.0046) ccw
  arc A336 (22.9631, -9.6526) -> (23.5464, -9.0779) centre (18.7439, -4.7871) ccw
  arc A337 (22.2541, -8.565) -> (22.2845, -9.3832) centre (28.6919, -8.7355) ccw
  arc A338 (22.3149, -7.9272) -> (22.2541, -8.565) centre (26.8603, -8.6825) ccw
  arc A339 (22.4031, -7.5531) -> (22.3149, -7.9272) centre (25.0601, -8.3772) ccw
  arc A340 (22.4332, -7.4675) -> (22.4031, -7.5531) centre (23.3923, -7.8522) ccw
  arc A341 (22.4332, -7.4675) -> (22.1673, -6.8364) centre (21.9304, -7.3078) ccw
  line L44 (22.1673, -6.8364) -> (22.1666, -6.8377)
  arc A342 (22.1666, -6.8377) -> (22.1546, -6.8303) centre (21.8828, -7.2824) ccw
  arc A343 (22.1546, -6.8303) -> (22.1417, -6.8244) centre (21.9304, -7.3078) ccw
  line L45 (22.1417, -6.8244) -> (22.1424, -6.8232)
  arc A344 (22.1424, -6.8232) -> (21.4702, -6.9538) centre (21.8828, -7.2824) ccw
  arc A345 (21.4158, -7.0264) -> (21.4702, -6.9538) centre (20.6165, -6.3715) ccw
  arc A346 (21.1542, -7.3081) -> (21.4158, -7.0264) centre (19.2515, -5.2787) ccw
  arc A347 (20.6584, -7.7138) -> (21.1542, -7.3081) centre (17.9953, -3.9536) ccw
  arc A348 (19.9619, -8.1443) -> (20.6584, -7.7138) centre (16.9311, -2.4619) ccw
  arc A349 (19.5126, -6.9262) -> (19.3602, -7.7307) centre (25.7511, -8.525) ccw
  arc A350 (19.7138, -6.318) -> (19.5126, -6.9262) centre (23.9772, -8.0657) ccw
  arc A351 (19.8831, -5.9728) -> (19.7138, -6.318) centre (22.2901, -7.3675) ccw
  arc A352 (19.9315, -5.896) -> (19.8831, -5.9728) centre (20.7809, -6.4845) ccw
  arc A353 (19.9315, -5.896) -> (19.8126, -5.2216) centre (19.4769, -5.6285) ccw
  line L46 (19.8126, -5.2216) -> (19.8117, -5.2227)
  arc A354 (19.8117, -5.2227) -> (19.8016, -5.2128) centre (19.4361, -5.5931) ccw
  arc A355 (19.8016, -5.2128) -> (19.7904, -5.2043) centre (19.4769, -5.6285) ccw
  line L47 (19.7904, -5.2043) -> (19.7913, -5.2032)
  arc A356 (19.7913, -5.2032) -> (19.1069, -5.1809) centre (19.4361, -5.5931) ccw
  arc A357 (19.0377, -5.2396) -> (19.1069, -5.1809) centre (18.4042, -4.4233) ccw
  arc A358 (18.72, -5.456) -> (19.0377, -5.2396) centre (17.3166, -3.0541) ccw
  arc A359 (18.1463, -5.7413) -> (18.72, -5.456) centre (16.3868, -1.4827) ccw
  arc A360 (17.3715, -6.006) -> (18.1463, -5.7413) centre (15.6812, 0.2084) ccw
  arc A361 (17.2046, -4.7185) -> (16.877, -5.4688) centre (22.9309, -7.6653) ccw
  arc A362 (17.5361, -4.1702) -> (17.2046, -4.7185) centre (21.3037, -6.8229) ccw
  arc A363 (17.7779, -3.8714) -> (17.5361, -4.1702) centre (19.8143, -5.7667) ccw
  arc A364 (17.8422, -3.8073) -> (17.7779, -3.8714) centre (18.5393, -4.57) ccw
  arc A365 (17.8422, -3.8073) -> (17.8764, -3.1234) centre (17.4585, -3.4453) ccw
  line L48 (17.8764, -3.1234) -> (17.8752, -3.1242)
  arc A366 (17.8752, -3.1242) -> (17.8676, -3.1123) centre (17.4266, -3.4017) ccw
  arc A367 (17.8676, -3.1123) -> (17.8586, -3.1015) centre (17.4585, -3.4453) ccw
  line L49 (17.8586, -3.1015) -> (17.8597, -3.1006)
  arc A368 (17.8597, -3.1006) -> (17.1974, -2.9266) centre (17.4266, -3.4017) ccw
  arc A369 (17.1169, -2.9685) -> (17.1974, -2.9266) centre (16.6809, -2.0316) ccw
  arc A370 (16.759, -3.1088) -> (17.1169, -2.9685) centre (15.9253, -0.4548) ccw
  arc A371 (16.1362, -3.2592) -> (16.759, -3.1088) centre (15.3684, 1.2841) ccw
  arc A372 (15.3219, -3.3448) -> (16.1362, -3.2592) centre (15.0568, 3.0898) ccw
  arc A373 (15.4457, -2.0525) -> (14.9593, -2.7111) centre (20.3727, -6.1997) ccw
  arc A374 (15.8909, -1.5917) -> (15.4457, -2.0525) centre (18.9737, -5.0163) ccw
  arc A375 (16.1931, -1.3542) -> (15.8909, -1.5917) centre (17.7567, -3.6551) ccw
  arc A376 (16.27, -1.306) -> (16.1931, -1.3542) centre (16.78, -2.2048) ccw
  arc A377 (16.27, -1.306) -> (16.4555, -0.6468) centre (15.9765, -0.8677) ccw
  line L50 (16.4555, -0.6468) -> (16.4542, -0.6474)
  arc A378 (16.4542, -0.6474) -> (16.4495, -0.6341) centre (15.9551, -0.8181) ccw
  arc A379 (16.4495, -0.6341) -> (16.4431, -0.6215) centre (15.9765, -0.8677) ccw
  line L51 (16.4431, -0.6215) -> (16.4444, -0.621)
  arc A380 (16.4444, -0.621) -> (15.8374, -0.3039) centre (15.9551, -0.8181) ccw
  arc A381 (15.7496, -0.3268) -> (15.8374, -0.3039) centre (15.533, 0.6835) ccw
  arc A382 (15.3694, -0.384) -> (15.7496, -0.3268) centre (15.1472, 2.389) ccw
  arc A383 (14.7288, -0.392) -> (15.3694, -0.384) centre (14.9912, 4.2082) ccw
  arc A384 (13.9159, -0.2943) -> (14.7288, -0.392) centre (15.0893, 6.038) ccw
  arc A385 (14.3241, 0.9381) -> (13.7033, 0.4042) centre (18.2047, -4.2015) ccw
  arc A386 (14.8607, 1.2882) -> (14.3241, 0.9381) centre (17.1042, -2.7365) ccw
  arc A387 (15.2082, 1.4525) -> (14.8607, 1.2882) centre (16.2205, -1.1386) ccw
  arc A388 (15.2939, 1.4824) -> (15.2082, 1.4525) centre (15.5911, 0.4927) ccw
  arc A389 (15.2939, 1.4824) -> (15.6214, 2.0838) centre (15.1053, 1.975) ccw
  line L52 (15.6214, 2.0838) -> (15.62, 2.0835)
  arc A390 (15.62, 2.0835) -> (15.6183, 2.0975) centre (15.0954, 2.0281) ccw
  arc A391 (15.6183, 2.0975) -> (15.6149, 2.1112) centre (15.1053, 1.975) ccw
  line L53 (15.6149, 2.1112) -> (15.6163, 2.1114)
  arc A392 (15.6163, 2.1114) -> (15.0951, 2.5556) centre (15.0954, 2.0281) ccw
  arc A393 (15.0044, 2.5528) -> (15.0951, 2.5556) centre (15.018, 3.5861) ccw
  arc A394 (14.6211, 2.5817) -> (15.0044, 2.5528) centre (15.0214, 5.3346) ccw
  arc A395 (13.9947, 2.7164) -> (14.6211, 2.5817) centre (15.2742, 7.1429) ccw
  arc A396 (13.2239, 2.9925) -> (13.9947, 2.7164) centre (15.7769, 8.905) ccw
  arc A397 (13.8961, 4.1032) -> (13.1721, 3.7208) centre (16.5358, -1.771) ccw
  arc A398 (14.4971, 4.3252) -> (13.8961, 4.1032) centre (15.7888, -0.0978) ccw
  arc A399 (14.8725, 4.408) -> (14.4971, 4.3252) centre (15.2829, 1.6566) ccw
  arc A400 (14.9627, 4.4181) -> (14.8725, 4.408) centre (15.0322, 3.3871) ccw
  arc A401 (14.9627, 4.4181) -> (15.4159, 4.9315) centre (14.8884, 4.9403) ccw
  line L54 (15.4159, 4.9315) -> (15.4144, 4.9315)
  arc A402 (15.4144, 4.9315) -> (15.4159, 4.9456) centre (14.8907, 4.9943) ccw
  arc A403 (15.4159, 4.9456) -> (15.4156, 4.9597) centre (14.8884, 4.9403) ccw
  line L55 (15.4156, 4.9597) -> (15.417, 4.9596)
  arc A404 (15.417, 4.9596) -> (15.0077, 5.5086) centre (14.8907, 4.9943) ccw
  arc A405 (14.9186, 5.5261) -> (15.0077, 5.5086) centre (15.1619, 6.5304) ccw
  arc A406 (14.5514, 5.6396) -> (14.9186, 5.5261) centre (15.5543, 8.2344) ccw
  arc A407 (13.9707, 5.9103) -> (14.5514, 5.6396) centre (16.2031, 9.9411) ccw
  arc A408 (13.2806, 6.351) -> (13.9707, 5.9103) centre (17.0853, 11.5471) ccw
  arc A409 (14.1832, 7.2843) -> (13.3922, 7.0726) centre (15.4495, 0.9699) ccw
  arc A410 (14.8185, 7.3669) -> (14.1832, 7.2843) centre (15.0936, 2.7674) ccw
  arc A411 (15.2029, 7.3641) -> (14.8185, 7.3669) centre (14.9907, 4.5904) ccw
  arc A412 (15.2931, 7.3539) -> (15.2029, 7.3641) centre (15.1314, 6.3332) ccw
  arc A413 (15.2931, 7.3539) -> (15.8491, 7.7536) centre (15.3369, 7.8795) ccw
  line L56 (15.8491, 7.7536) -> (15.8477, 7.7539)
  arc A414 (15.8477, 7.7539) -> (15.8523, 7.7673) centre (15.351, 7.9316) ccw
  arc A415 (15.8523, 7.7673) -> (15.8551, 7.7811) centre (15.3369, 7.8795) ccw
  line L57 (15.8551, 7.7811) -> (15.8565, 7.7808)
  arc A416 (15.8565, 7.7808) -> (15.5796, 8.4071) centre (15.351, 7.9316) ccw
  arc A417 (15.4967, 8.4439) -> (15.5796, 8.4071) centre (15.9573, 9.3689) ccw
  arc A418 (15.1638, 8.6363) -> (15.4967, 8.4439) centre (16.719, 10.9428) ccw
  arc A419 (14.658, 9.0294) -> (15.1638, 8.6363) centre (17.7313, 12.4624) ccw
  arc A420 (14.0833, 9.6126) -> (14.658, 9.0294) centre (18.9488, 13.8318) ccw
  arc A421 (15.1709, 10.3217) -> (14.3527, 10.2913) centre (15.0004, 3.8838) ccw
  arc A422 (15.8086, 10.2608) -> (15.1709, 10.3217) centre (15.0534, 5.7154) ccw
  arc A423 (16.1828, 10.1726) -> (15.8086, 10.2608) centre (15.3587, 7.5156) ccw
  arc A424 (16.2684, 10.1425) -> (16.1828, 10.1726) centre (15.8837, 9.1835) ccw
  arc A425 (16.2684, 10.1425) -> (16.8995, 10.4085) centre (16.4281, 10.6453) ccw
  line L58 (16.8995, 10.4085) -> (16.8982, 10.4092)
  arc A426 (16.8982, 10.4092) -> (16.9056, 10.4212) centre (16.4535, 10.6929) ccw
  arc A427 (16.9056, 10.4212) -> (16.9115, 10.434) centre (16.4281, 10.6453) ccw
  line L59 (16.9115, 10.434) -> (16.9127, 10.4333)
  arc A428 (16.9127, 10.4333) -> (16.7821, 11.1056) centre (16.4535, 10.6929) ccw
  arc A429 (16.7095, 11.1599) -> (16.7821, 11.1056) centre (17.3644, 11.9593) ccw
  arc A430 (16.4278, 11.4215) -> (16.7095, 11.1599) centre (18.4572, 13.3242) ccw
  arc A431 (16.0221, 11.9174) -> (16.4278, 11.4215) centre (19.7823, 14.5805) ccw
  arc A432 (15.5916, 12.6139) -> (16.0221, 11.9174) centre (21.274, 15.6446) ccw
  arc A433 (16.8097, 13.0631) -> (16.0052, 13.2155) centre (15.2109, 6.8246) ccw
  arc A434 (17.4179, 12.8619) -> (16.8097, 13.0631) centre (15.6702, 8.5985) ccw
  arc A435 (17.7631, 12.6926) -> (17.4179, 12.8619) centre (16.3684, 10.2856) ccw
  arc A436 (17.8399, 12.6443) -> (17.7631, 12.6926) centre (17.2514, 11.7949) ccw
  arc A437 (17.8399, 12.6443) -> (18.5143, 12.7631) centre (18.1074, 13.0989) ccw
  line L60 (18.5143, 12.7631) -> (18.5132, 12.7641)
  arc A438 (18.5132, 12.7641) -> (18.5231, 12.7741) centre (18.1428, 13.1397) ccw
  arc A439 (18.5231, 12.7741) -> (18.5316, 12.7853) centre (18.1074, 13.0989) ccw
  line L61 (18.5316, 12.7853) -> (18.5327, 12.7844)
  arc A440 (18.5327, 12.7844) -> (18.555, 13.4688) centre (18.1428, 13.1397) ccw
  arc A441 (18.4963, 13.538) -> (18.555, 13.4688) centre (19.3126, 14.1716) ccw
  arc A442 (18.2799, 13.8557) -> (18.4963, 13.538) centre (20.6818, 15.2591) ccw
  arc A443 (17.9946, 14.4294) -> (18.2799, 13.8557) centre (22.2532, 16.189) ccw
  arc A444 (17.7299, 15.2042) -> (17.9946, 14.4294) centre (23.9443, 16.8945) ccw
  arc A445 (19.0174, 15.3712) -> (18.2671, 15.6988) centre (16.0706, 9.6448) ccw
  arc A446 (19.5657, 15.0396) -> (19.0174, 15.3712) centre (16.913, 11.2721) ccw
  arc A447 (19.8645, 14.7978) -> (19.5657, 15.0396) centre (17.9692, 12.7615) ccw
  arc A448 (19.9286, 14.7336) -> (19.8645, 14.7978) centre (19.1658, 14.0364) ccw
  arc A449 (19.9286, 14.7336) -> (20.6125, 14.6994) centre (20.2906, 15.1172) ccw
  line L62 (20.6125, 14.6994) -> (20.6117, 14.7005)
  arc A450 (20.6117, 14.7005) -> (20.6236, 14.7081) centre (20.3342, 15.1491) ccw
  arc A451 (20.6236, 14.7081) -> (20.6344, 14.7172) centre (20.2906, 15.1172) ccw
  line L63 (20.6344, 14.7172) -> (20.6353, 14.716)
  arc A452 (20.6353, 14.716) -> (20.8093, 15.3783) centre (20.3342, 15.1491) ccw
  arc A453 (20.7674, 15.4588) -> (20.8093, 15.3783) centre (21.7043, 15.8949) ccw
  arc A454 (20.6271, 15.8168) -> (20.7674, 15.4588) centre (23.2811, 16.6505) ccw
  arc A455 (20.4767, 16.4395) -> (20.6271, 15.8168) centre (25.02, 17.2074) ccw
  arc A456 (20.3911, 17.2538) -> (20.4767, 16.4395) centre (26.8257, 17.5189) ccw
  arc A457 (21.6834, 17.1301) -> (21.0248, 17.6165) centre (17.5362, 12.203) ccw
  arc A458 (22.1442, 16.6849) -> (21.6834, 17.1301) centre (18.7196, 13.602) ccw
  arc A459 (22.3817, 16.3826) -> (22.1442, 16.6849) centre (20.0808, 14.8191) ccw
  arc A460 (22.4299, 16.3057) -> (22.3817, 16.3826) centre (21.5311, 15.7958) ccw
  arc A461 (22.4299, 16.3057) -> (23.0891, 16.1202) centre (22.8682, 16.5992) ccw
  line L64 (23.0891, 16.1202) -> (23.0885, 16.1215)
  arc A462 (23.0885, 16.1215) -> (23.1018, 16.1263) centre (22.9178, 16.6206) ccw
  arc A463 (23.1018, 16.1263) -> (23.1144, 16.1327) centre (22.8682, 16.5992) ccw
  line L65 (23.1144, 16.1327) -> (23.1149, 16.1314)
  arc A464 (23.1149, 16.1314) -> (23.4319, 16.7383) centre (22.9178, 16.6206) ccw
  arc A465 (23.409, 16.8262) -> (23.4319, 16.7383) centre (24.4194, 17.0428) ccw
  arc A466 (23.3519, 17.2063) -> (23.409, 16.8262) centre (26.1249, 17.4286) ccw
  arc A467 (23.3439, 17.8469) -> (23.3519, 17.2063) centre (27.9441, 17.5845) ccw
  arc A468 (23.4416, 18.6599) -> (23.3439, 17.8469) centre (29.7739, 17.4865) ccw
  arc A469 (24.674, 18.2516) -> (24.1401, 18.8724) centre (19.5344, 14.371) ccw
  arc A470 (25.0241, 17.7151) -> (24.674, 18.2516) centre (20.9994, 15.4715) ccw
  arc A471 (25.1884, 17.3675) -> (25.0241, 17.7151) centre (22.5973, 16.3552) ccw
  arc A472 (25.2183, 17.2819) -> (25.1884, 17.3675) centre (24.2286, 16.9847) ccw
  arc A473 (25.2183, 17.2819) -> (25.8196, 16.9543) centre (25.7109, 17.4705) ccw
  line L66 (25.8196, 16.9543) -> (25.8194, 16.9557)
  arc A474 (25.8194, 16.9557) -> (25.8334, 16.9574) centre (25.764, 17.4803) ccw
  arc A475 (25.8334, 16.9574) -> (25.8471, 16.9609) centre (25.7109, 17.4705) ccw
  line L67 (25.8471, 16.9609) -> (25.8473, 16.9594)
  arc A476 (25.8473, 16.9594) -> (26.2915, 17.4807) centre (25.764, 17.4803) ccw
  arc A477 (26.2887, 17.5714) -> (26.2915, 17.4807) centre (27.322, 17.5577) ccw
  arc A478 (26.3176, 17.9547) -> (26.2887, 17.5714) centre (29.0705, 17.5543) ccw
  arc A479 (26.4523, 18.5811) -> (26.3176, 17.9547) centre (30.8788, 17.3016) ccw
  arc A480 (26.7284, 19.3519) -> (26.4523, 18.5811) centre (32.6409, 16.7988) ccw
  arc A481 (27.8391, 18.6796) -> (27.4567, 19.4036) centre (21.9649, 16.0399) ccw
  arc A482 (28.0611, 18.0786) -> (27.8391, 18.6796) centre (23.6381, 16.7869) ccw
  arc A483 (28.1439, 17.7032) -> (28.0611, 18.0786) centre (25.3925, 17.2929) ccw
  arc A484 (28.154, 17.613) -> (28.1439, 17.7032) centre (27.123, 17.5436) ccw
  arc A485 (28.154, 17.613) -> (28.6674, 17.1599) centre (28.6762, 17.6873) ccw
  line L68 (28.6674, 17.1599) -> (28.6674, 17.1613)
  arc A486 (28.6674, 17.1613) -> (28.6815, 17.1598) centre (28.7302, 17.6851) ccw
  arc A487 (28.6815, 17.1598) -> (28.6956, 17.1602) centre (28.6762, 17.6873) ccw
  line L69 (28.6956, 17.1602) -> (28.6955, 17.1587)
  arc A488 (28.6955, 17.1587) -> (29.2445, 17.568) centre (28.7302, 17.6851) ccw
  arc A489 (29.262, 17.6571) -> (29.2445, 17.568) centre (30.2663, 17.4139) ccw
  arc A490 (29.3755, 18.0244) -> (29.262, 17.6571) centre (31.9703, 17.0215) ccw
  arc A491 (29.6462, 18.6051) -> (29.3755, 18.0244) centre (33.677, 16.3727) ccw
  arc A492 (30.0869, 19.2951) -> (29.6462, 18.6051) centre (35.283, 15.4904) ccw
  arc A493 (-7.9473, 18.9358) -> (-8.5899, 18.8537) centre (-7.2557, 10.9657) ccw
  arc A494 (-11.3369, 17.8464) -> (-11.8803, 17.4936) centre (-7.2557, 10.9657) ccw
  arc A495 (-13.9181, 15.3942) -> (-14.2546, 14.8406) centre (-7.2557, 10.9657) ccw
  arc A496 (-15.1798, 12.0649) -> (-15.2428, 11.4201) centre (-7.2557, 10.9657) ccw
  arc A497 (-14.872, 8.5179) -> (-14.649, 7.9097) centre (-7.2557, 10.9657) ccw
  arc A498 (-13.0557, 5.4557) -> (-12.5908, 5.0045) centre (-7.2557, 10.9657) ccw
  arc A499 (-10.0906, 3.4849) -> (-9.476, 3.28) centre (-7.2557, 10.9657) ccw
  arc A500 (-6.5641, 2.9957) -> (-5.9214, 3.0778) centre (-7.2557, 10.9657) ccw
  arc A501 (-3.1745, 4.085) -> (-2.6311, 4.4378) centre (-7.2557, 10.9657) ccw
  arc A502 (-0.5932, 6.5372) -> (-0.2567, 7.0908) centre (-7.2557, 10.9657) ccw
  arc A503 (0.6684, 9.8665) -> (0.7314, 10.5113) centre (-7.2557, 10.9657) ccw
  arc A504 (0.3606, 13.4135) -> (0.1376, 14.0217) centre (-7.2557, 10.9657) ccw
  arc A505 (-1.4557, 16.4757) -> (-1.9205, 16.9269) centre (-7.2557, 10.9657) ccw
  arc A506 (-4.4207, 18.4466) -> (-5.0353, 18.6514) centre (-7.2557, 10.9657) ccw
  arc A507 (16.877, -5.4688) -> (17.3715, -6.006) centre (28.1558, 4.4199) ccw
  arc A508 (19.3602, -7.7307) -> (19.9619, -8.1443) centre (28.1558, 4.4199) ccw
  arc A509 (22.2845, -9.3832) -> (22.9631, -9.6526) centre (28.1558, 4.4199) ccw
  arc A510 (25.5032, -10.3437) -> (26.2247, -10.4553) centre (28.1558, 4.4199) ccw
  arc A511 (28.8549, -10.5638) -> (29.5832, -10.512) centre (28.1558, 4.4199) ccw
  arc A512 (32.1716, -10.0325) -> (32.8701, -9.82) centre (28.1558, 4.4199) ccw
  arc A513 (35.2868, -8.7766) -> (35.9206, -8.414) centre (28.1558, 4.4199) ccw
  arc A514 (38.0446, -6.8589) -> (38.5817, -6.3644) centre (28.1558, 4.4199) ccw
  arc A515 (40.3064, -4.3757) -> (40.72, -3.774) centre (28.1558, 4.4199) ccw
  arc A516 (41.959, -1.4514) -> (42.2283, -0.7728) centre (28.1558, 4.4199) ccw
  arc A517 (42.9194, 1.7673) -> (43.031, 2.4888) centre (28.1558, 4.4199) ccw
  arc A518 (43.1395, 5.119) -> (43.0878, 5.8473) centre (28.1558, 4.4199) ccw
  arc A519 (42.6083, 8.4357) -> (42.3958, 9.1342) centre (28.1558, 4.4199) ccw
  arc A520 (41.3523, 11.551) -> (40.9897, 12.1847) centre (28.1558, 4.4199) ccw
  arc A521 (39.4347, 14.3087) -> (38.9401, 14.8458) centre (28.1558, 4.4199) ccw
  arc A522 (36.9514, 16.5705) -> (36.3498, 16.9841) centre (28.1558, 4.4199) ccw
  arc A523 (34.0272, 18.2231) -> (33.3485, 18.4924) centre (28.1558, 4.4199) ccw
  arc A524 (30.8085, 19.1835) -> (30.0869, 19.2951) centre (28.1558, 4.4199) ccw
  arc A525 (27.4567, 19.4036) -> (26.7284, 19.3519) centre (28.1558, 4.4199) ccw
  arc A526 (24.1401, 18.8724) -> (23.4416, 18.6599) centre (28.1558, 4.4199) ccw
  arc A527 (21.0248, 17.6165) -> (20.3911, 17.2538) centre (28.1558, 4.4199) ccw
  arc A528 (18.2671, 15.6988) -> (17.7299, 15.2042) centre (28.1558, 4.4199) ccw
  arc A529 (16.0052, 13.2155) -> (15.5916, 12.6139) centre (28.1558, 4.4199) ccw
  arc A530 (14.3527, 10.2913) -> (14.0833, 9.6126) centre (28.1558, 4.4199) ccw
  arc A531 (13.3922, 7.0726) -> (13.2806, 6.351) centre (28.1558, 4.4199) ccw
  arc A532 (13.1721, 3.7208) -> (13.2239, 2.9925) centre (28.1558, 4.4199) ccw
  arc A533 (13.7033, 0.4042) -> (13.9159, -0.2943) centre (28.1558, 4.4199) ccw
  arc A534 (14.9593, -2.7111) -> (15.3219, -3.3448) centre (28.1558, 4.4199) ccw
  point P0 (-15.1798, 12.0649)
  point P1 (-15.231, 11.5938)
  point P2 (-14.872, 8.5179)
  point P3 (-14.649, 7.9097)
  point P4 (-13.0557, 5.4557)
  point P5 (-10.0906, 3.4849)
  point P6 (-6.5641, 2.9957)
  point P7 (-5.9214, 3.0778)
  point P8 (-3.1745, 4.085)
  point P9 (-2.6311, 4.4378)
  point P10 (-0.5932, 6.5372)
  point P11 (-0.2567, 7.0908)
  point P12 (0.6684, 9.8665)
  point P13 (0.7314, 10.5113)
  point P14 (0.3606, 13.4135)
  point P15 (0.1376, 14.0217)
  point P16 (-1.4557, 16.4757)
  point P17 (-1.9205, 16.9269)
  point P18 (-4.4207, 18.4466)
  point P19 (-5.0353, 18.6514)
  point P20 (-7.9473, 18.9358)
  point P21 (-11.3369, 17.8464)
  point P22 (-11.8803, 17.4936)
  point P23 (-13.9181, 15.3942)
  point P24 (-14.2546, 14.8406)
  point P25 (30.8085, 19.1835)
  point P26 (27.4567, 19.4036)
  point P27 (26.7284, 19.3519)
  point P28 (21.0248, 17.6165)
  point P29 (18.2671, 15.6988)
  point P30 (17.7299, 15.2042)
  point P31 (16.0052, 13.2155)
  point P32 (15.5916, 12.6139)
  point P33 (14.3527, 10.2913)
  point P34 (14.0833, 9.6126)
  point P35 (13.3922, 7.0726)
  point P36 (13.1721, 3.7208)
  point P37 (13.2239, 2.9925)
  point P38 (13.7033, 0.4042)
  point P39 (13.9159, -0.2943)
  point P40 (14.9593, -2.7111)
  point P41 (15.3219, -3.3448)
  point P42 (16.877, -5.4688)
  point P43 (17.3715, -6.006)
  point P44 (19.3602, -7.7307)
  point P45 (22.2845, -9.3832)
  point P46 (22.9631, -9.6526)
  point P47 (25.5032, -10.3437)
  point P48 (32.1716, -10.0325)
  point P49 (35.2868, -8.7766)
  point P50 (38.0446, -6.8589)
  point P51 (38.5817, -6.3644)
  point P52 (40.72, -3.774)
  point P53 (41.959, -1.4514)
  point P54 (42.2283, -0.7728)
  point P55 (42.9194, 1.7673)
  point P56 (43.031, 2.4888)
  point P57 (43.1395, 5.119)
  point P58 (43.0878, 5.8473)
  point P59 (42.6083, 8.4357)
  point P60 (41.3523, 11.551)
  point P61 (39.4347, 14.3087)
  point P62 (38.9401, 14.8458)
  point P63 (36.9514, 16.5705)
  point P64 (34.0272, 18.2231)
  constraints: 1010 point on circle, 507 centre point, 140 end point, 84 other